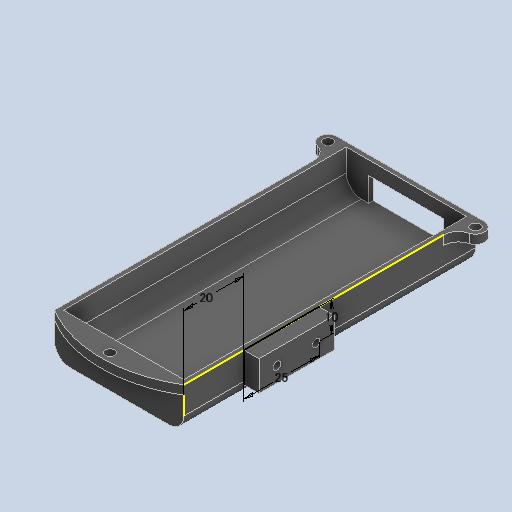
# Autodesk Inventor part: handle_monitor_case_under
Saved by Autodesk Inventor 2026.1 (Build 301233020, 233B)
## iProperties
Created: 2026-02-03
Part Number: handle_monitor_case_under
Material: 一般
Document SubType Name: Modeling
Designer: hibik
Density: 1 g/cm^3
Appearance: 既定
Author: hibik
Autodesk Inventor part; units mm, degrees
ref_plane "YZ Plane" through (0, 0, 0) normal (1, 0, 0) x (0, 1, 0)
ref_plane "XZ Plane" through (0, 0, 0) normal (0, 1, 0) x (-1, 0, 0)
sketch "スケッチ1" plane through (0, 0, 0) normal (0, 1, 0) x (-1, 0, 0)
  line L0 (21.5, -48.5) -> (-21.5, -48.5)
  line L1 (-21.5, -48.5) -> (-21.5, 48.5)
  line L2 (-21.5, 48.5) -> (21.5, 48.5)
  line L3 (21.5, 48.5) -> (21.5, -48.5)
  line L4 (21.5, -48.5) -> (-21.5, 48.5) construction
  line L5 (-21.5, -48.5) -> (21.5, 48.5) construction
  point P0 (0, 0)
  dimension "d0" = 43
  dimension "d1" = 97
  constraints: 12 end point, 2 midpoint, 2 parallel, 1 horizontal, 1 perpendicular
  measures "d0" distance of L1.end L2.end
  measures "d1" distance of L0.end L1.end
extrude "押し出し1" add sketch "スケッチ1" along normal blind 14
shell "シェル1" thickness 1.5 removed faces 1 at (-7.1667, 14, -16.1667)
fillet "フィレット1" radius 5 4 edges at (-21.5, 0, 0) (21.5, 0, 0) (-20, 1.5, 0) (20, 1.5, 0)
sketch "スケッチ2" plane through (21.5, 14, -48.5) normal (0, 0, -1) x (-1, 0, 0)
  arc A0 (1.5, -7.5) -> (6.5, -12.5) centre (6.5, -7.5) ccw projected
  line L0 (1.5, -7.5) -> (1.5, 0) projected
  line L1 (41.5, 0) -> (1.5, 0) projected
  line L2 (41.5, -7.5) -> (41.5, 0) projected
  arc A1 (36.5, -12.5) -> (41.5, -7.5) centre (36.5, -7.5) ccw projected
  line L3 (6.5, -12.5) -> (36.5, -12.5) projected
  line L4 (1.5, -4.5) -> (41.5, -4.5)
  line L5 (9, -4.5) -> (34, -4.5)
  line L6 (34, -4.5) -> (34, -12.5)
  line L7 (34, -12.5) -> (9, -12.5)
  line L8 (9, -12.5) -> (9, -4.5)
  point P0 (21.5, -14)
  point P1 (21.5, -4.5)
  point P2 (9, -12.5)
  dimension "d8" = 8
  dimension "d9" = 25
  constraints: 10 end point, 4 point on line, 2 horizontal, 2 midpoint, 2 parallel, 1 perpendicular
  measures "d8" distance between parallel lines of L3 L4
  measures "d9" distance between parallel lines of L6 L8
extrude "押し出し2" cut sketch "スケッチ2" against normal up to surface (1.5 mm away) contours L8 L4 L6 L3
sketch "スケッチ3" plane through (0, 0, 0) normal (0, -1, 0) x (1, 0, 0)
  circle A0 centre (0, 51.5) radius 3
  circle A1 centre (24.5, -45.5) radius 3
  circle A2 centre (-24.5, -45.5) radius 3
  line L0 (-21.5, 48.5) -> (-21.5, -48.5) projected
  line L1 (16.5, -48.5) -> (-16.5, -48.5) projected
  line L2 (21.5, -48.5) -> (21.5, 48.5) projected
  line L3 (-16.5, 48.5) -> (16.5, 48.5) projected
  line L4 (-24.5, -48.5) -> (24.5, -48.5)
  arc A3 (21.5, 48.5) -> (-21.5, 48.5) centre (0, 12.9792) ccw
  line L5 (-21.5, 48.5) -> (-16.5, 48.5) projected
  line L6 (16.5, 48.5) -> (21.5, 48.5) projected
  circle A4 centre (0, 51.5) radius 1.6
  circle A5 centre (24.5, -45.5) radius 1.6
  circle A6 centre (-24.5, -45.5) radius 1.6
  point P0 (0, 0)
  point P1 (-21.5, -45.5)
  point P2 (21.5, -45.5)
  dimension "d11" = 6
  dimension "d12" = 6
  dimension "d10" = 6
  dimension "d13" = 3.2
  dimension "d14" = 3.2
  dimension "d15" = 3.2
  constraints: 5 centre point, 3 coincident, 2 end point, 2 horizontal, 2 point on circle, 2 tangent, 2 vertical, 1 collinear, 1 vertical alignment, 6 other
  measures "d10" diameter of A0
  measures "d13" diameter of A4
  measures "d14" diameter of A5
  measures "d15" diameter of A6
extrude "押し出し3" add sketch "スケッチ3" against normal up to surface (14 mm away) contours A0 | A0 A3 L6 L3 | A0 L3 L5 A3 | A1 | A1 L4 L2 | A2 | L0 L4 A2
extrude "押し出し4" cut sketch "スケッチ3" against normal blind 11 contours A0 | A0 A3 L6 L3 | A0 L3 L5 A3 | A1 | A1 L4 L2 | A2 | L0 L4 A2 | A4 | A6
fillet "フィレット2" radius 5 2 edges at (-21.5, 12.5, -45.5) (21.5, 12.5, -45.5)
sketch "スケッチ4" plane through (21.5, 5, 48.5) normal (1, 0, 0) x (0, 0, -1)
  line L0 (20, 9) -> (45, 9)
  line L1 (45, 9) -> (45, -1)
  line L2 (45, -1) -> (20, -1)
  line L3 (20, -1) -> (20, 9)
  line L4 (0, 9) -> (86.254, 9) projected
  line L5 (0, 0) -> (0, 6) projected
  point P0 (48.5, -5)
  dimension "d21" = 25
  dimension "d22" = 10
  dimension "d23" = 20
  constraints: 8 end point, 2 parallel, 1 horizontal, 1 perpendicular, 1 point on line
  measures "d21" distance of L1.end L2.end
  measures "d22" distance of L0.end L1.end
  measures "d23" distance between parallel lines of L5 L3
extrude "押し出し5" add sketch "スケッチ4" along normal blind 5
sketch "スケッチ5" plane through (26.5, 5, 48.5) normal (1, 0, 0) x (0, 0, -1)
  circle A0 centre (26, 4) radius 1.3
  circle A1 centre (39, 4) radius 1.3
  line L0 (20, 9) -> (20, -1) projected
  line L1 (45, -1) -> (45, 9) projected
  point P0 (48.5, -5)
  point P1 (20, 4)
  dimension "d26" = 2.6
  dimension "d27" = 2.6
  dimension "d28" = 6
  dimension "d29" = 6
  constraints: 2 centre point, 2 horizontal alignment, 1 midpoint
  measures "d26" diameter of A0
  measures "d27" diameter of A1
  measures "d28" distance from line of L0 A0.centre
  measures "d29" distance from line of L1 A1.centre
ref_plane "作業平面1" through (18.75, 8.39, -7.25) normal (1, 0, 0) x (0, 1, 0)
extrude "押し出し6" cut sketch "スケッチ5" against normal up to surface (7.75 mm away)
sketch "スケッチ6" plane through (21.5, 4, 28.5) normal (0, 0, 1) x (1, 0, 0)
  arc A0 (-5, -4) -> (0, 1) centre (-5, 1) ccw projected
  line L0 (0, 0) -> (5, 0) projected
  line L1 (0, 1) -> (0, 0) projected
  line L2 (0, 0) -> (-0.101, 0)
  point P0 (-21.5, -4)
  constraints: 2 end point, 1 horizontal, 1 point on circle
extrude "押し出し7" add sketch "スケッチ6" against normal up to surface (25 mm away)
